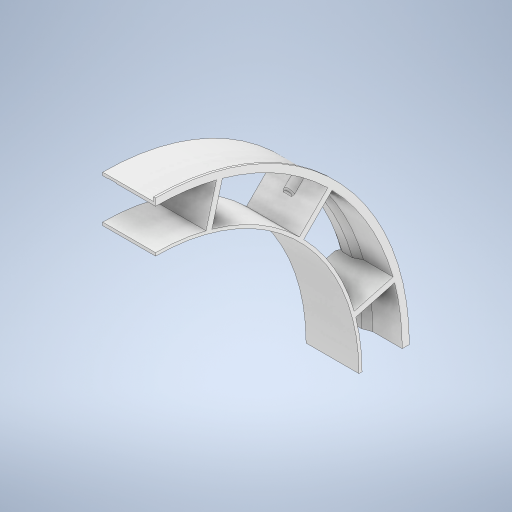
# Autodesk Inventor part: Abstandshalter_Röhre_Neu
Saved by Autodesk Inventor 2023 (Build 270158000, 158)
## iProperties
Created: 2023-03-14
Part Number: Abstandshalter_Röhre_Neu
Material: Generisch
Document SubType Name: Modeling
Designer: prigge
Density: 1 g/cm^3
Appearance: Glatt - Weiß
Author: prigge
Autodesk Inventor part; units mm, degrees
ref_plane "YZ Plane" through (0, 0, 0) normal (1, 0, 0) x (0, 1, 0)
sketch "Skizze1" plane through (0, 0, 0) normal (1, 0, 0) x (0, 1, 0)
  arc A0 (0, -200) -> (200, 0) centre (0, 0) ccw
  arc A1 (0, -203) -> (203, 0) centre (0, 0) ccw
  line L0 (203, 0) -> (200, 0)
  line L1 (0, -200) -> (0, -203)
  line L2 (0, -294.0512) -> (0, 49.0085) projected
  line L3 (-49.0085, 0) -> (294.0512, 0) projected
  dimension "d0" = 200
  dimension "d1" = 3
  constraints: 4 end point, 4 point on circle, 2 centre point, 2 coincident, 2 point on line, 1 horizontal, 1 perpendicular
  measures "d0" radius of A0
  measures "d1" distance of L1.start L1.end
extrude "Extrusion1" add sketch "Skizze1" against normal blind 52 contours A0 L0 A1 L1
sketch "Skizze2" plane through (0, 0, 0) normal (1, 0, 0) x (0, 1, 0)
  arc A0 (0, -242.5) -> (242.5, 0) centre (0, 0) ccw
  arc A1 (0, -245.5) -> (245.5, 0) centre (0, 0) ccw
  line L0 (245.5, 0) -> (242.5, 0)
  line L1 (0, -242.5) -> (0, -245.5)
  line L2 (0, -354.8894) -> (0, 59.1482) projected
  line L3 (-59.1482, 0) -> (354.8894, 0) projected
  dimension "d4" = 3
  dimension "d5" = 245.5
  constraints: 4 end point, 4 point on circle, 2 centre point, 2 coincident, 2 point on line, 1 horizontal, 1 perpendicular
  measures "d4" distance of L1.start L1.end
  measures "d5" radius of A1
extrude "Extrusion2" add sketch "Skizze2" against normal blind 52 contours A0 L0 A1 L1
sketch "Skizze3" plane through (0, 0, 0) normal (1, 0, 0) x (0, 1, 0)
  arc A0 (0, -249.5) -> (249.5, 0) centre (0, 0) ccw
  arc A1 (0, -245.5) -> (245.5, 0) centre (0, 0) ccw projected
  line L0 (242.5, 0) -> (245.5, 0) projected
  arc A2 (0, -245.5) -> (245.5, 0) centre (0, 0) ccw
  line L1 (0, -245.5) -> (0, -249.5)
  line L2 (245.5, 0) -> (249.5, 0)
  dimension "d29" = 4
  constraints: 4 end point, 4 point on circle, 2 centre point, 2 coincident, 1 perpendicular, 1 vertical
  measures "d29" distance of L1.start L1.end
extrude "Extrusion3" add sketch "Skizze3" against normal blind 2
sketch "Skizze4" plane through (0, 0, 0) normal (1, 0, 0) x (0, 1, 0)
  line L0 (0, 0) -> (176.4231, -176.4231) construction
  arc A0 (0, -249.5) -> (249.5, 0) centre (0, 0) ccw projected
  line L1 (0, -362.132) -> (0, 60.3553) projected
  arc A1 (0, -203) -> (203, 0) centre (0, 0) ccw projected
  arc A2 (0, -242.5) -> (242.5, 0) centre (0, 0) ccw projected
  arc A3 (0, -203) -> (203, 0) centre (0, 0) ccw projected
  line L2 (145.6483, -141.4057) -> (173.5816, -169.339)
  arc A4 (0, -242.5) -> (242.5, 0) centre (0, 0) ccw projected
  line L3 (141.4057, -145.6483) -> (169.339, -173.5816)
  point P0 (169.339, -173.5816)
  point P1 (173.5816, -169.339)
  dimension "d11" = 45
  dimension "d12" = 3
  dimension "d13" = 3
  constraints: 6 end point, 5 point on circle
  measures "d11" angle of L1 L0
  measures "d12" distance between parallel lines of L0 L2
  measures "d13" distance between parallel lines of L0 L3
extrude "Extrusion4" add sketch "Skizze4" against normal up to surface (52 mm away) contours L3 A1 L2 A2
pattern_circular "Runde Anordnung1" count 2 over 30 about axis through (-10, 0, 0) along (1, 0, 0) of "Extrusion4"
ref_plane "Arbeitsebene1" through (0, 0, 0) normal (0, 0.7071068, 0.7071068) x (1, 0, 0)
mirror "Spiegeln1" about plane through (0, 0, 0) normal (0, 0.7071068, 0.7071068) of "Extrusion4", "Runde Anordnung1"
ref_plane "Arbeitsebene3" through (0, 171.4734, -171.4734) normal (0, 0.7071068, -0.7071068) x (1, 0, 0)
ref_plane "Arbeitsebene2" through (0, 0, 0) normal (0, 0.7071068, -0.7071068) x (1, 0, 0)
sketch "Skizze5" plane through (0, 171.4734, -171.4734) normal (0, 0.7071068, -0.7071068) x (1, 0, 0)
  circle A0 centre (-27, 0) radius 6
  line L0 (0, 246.9924) -> (0, -246.9924) projected
  circle A1 centre (-27, 0) radius 4
  line L1 (-62.4, 0) -> (10.4, 0) projected
  point P0 (0, 0)
  dimension "d21" = 27
  dimension "d22" = 8
  dimension "d23" = 12
  constraints: 2 centre point, 1 coincident, 1 point on line
  measures "d21" distance from line of L0 A0.centre
  measures "d22" diameter of A1
  measures "d23" diameter of A0
extrude "Extrusion5" add sketch "Skizze5" against normal blind 16
fillet "Rundung2" radius 2 4 edges at (-27, 155.917, -164.4023) (-27, 164.4023, -155.917) (-27, 162.281, -158.0384) (-27, 158.0384, -162.281)
sketch "Skizze9" plane through (0, 0, 0) normal (0, 1, 0) x (-1, 0, 0)
  line L0 (0, -242.5) -> (52, -242.5) projected
  line L1 (52, -245.5) -> (52, -242.5) projected
  line L2 (29, -242.5) -> (37, -239.5)
  line L3 (37, -239.5) -> (47, -239.5)
  line L4 (52, -245.5) -> (52, 0) projected
  line L5 (47, -239.5) -> (47, -242.5)
  line L6 (62.4, 0) -> (-10.4, 0) projected
  point P0 (0, 0)
  dimension "d38" = 3
  dimension "d39" = 5
  dimension "d40" = 18
  dimension "d41" = 10
  constraints: 6 end point, 2 perpendicular, 2 point on line
  measures "d38" distance of L3.end L5.end
  measures "d39" distance between parallel lines of L4 L5
  measures "d40" distance from line of L5 L2.start
  measures "d41" distance of L2.end L3.end
revolve "Umdrehung2" add sketch "Skizze9" angle 87 about axis through (-10, 0, 0) along (1, 0, 0)
sketch "Skizze10" plane through (0, 0, 0) normal (0, 1, 0) x (-1, 0, 0)
  line L0 (47, -242.5) -> (47, -239.5) projected
  line L1 (47, -239.5) -> (37, -239.5) projected
  line L2 (52, -245.5) -> (52, -242.5) projected
  line L3 (47, -240.8) -> (38.5, -240.8)
  line L4 (38.5, -240.8) -> (38.5, -243)
  line L5 (38.5, -243) -> (47, -243)
  line L6 (47, -243) -> (47, -240.8)
  line L7 (47, -242.5) -> (52, -242.5) projected
  line L8 (52, -245.5) -> (52, 0) projected
  arc A0 (47, -240.8) -> (52, -237.0283) centre (47, -235.6) ccw
  line L9 (52, -242.5) -> (52, -237.0283)
  line L10 (63.1578, 0) -> (-10.5263, 0) projected
  line L11 (47, -232.0975) -> (47, -239.5) projected
  point P0 (0, 0)
  dimension "d44" = 2.2
  dimension "d45" = 8.5
  dimension "d46" = 5.2
  dimension "d48" = 0.5
  constraints: 10 end point, 3 point on line, 2 parallel, 2 point on circle, 1 centre point, 1 collinear, 1 horizontal, 1 perpendicular
  measures "d44" distance of L3.end L4.end
  measures "d45" distance of L4.end L5.end
  measures "d46" radius of A0
  measures "d48" distance between parallel lines of L7 L5
revolve "Umdrehung3" cut sketch "Skizze10" angle 90 about axis through (-10, 0, 0) along (1, 0, 0)
fillet "Rundung3" radius 2 1 edges at (-47, 171.8269, -171.8269)
extrude "Extrusion6" cut sketch "Skizze5" along normal mid plane 26 contours L1 A1 | A1 L1
sketch "Skizze7" plane through (0, 0, 0) normal (1, 0, 0) x (0, 1, 0)
  line L0 (0, -242.5) -> (0, -249.5) projected
  circle A0 centre (0, -249.5) radius 2.5
  circle A1 centre (0, -242.5) radius 2.5
  line L1 (0, -203) -> (0, -200) projected
  circle A2 centre (0, -203) radius 2.5
  circle A3 centre (0, -200) radius 2.5
  line L2 (249.5, 0) -> (242.5, 0) projected
  circle A4 centre (249.5, 0) radius 2.5
  circle A5 centre (242.5, 0) radius 2.5
  arc A6 (196.838, -49.6368) -> (203, 0) centre (0, 0) ccw projected
  circle A7 centre (203, 0) radius 2.5
  arc A8 (0, -200) -> (200, 0) centre (0, 0) ccw projected
  circle A9 centre (200, 0) radius 2.5
  point P0 (201.5, -2)
  point P1 (201.5, 2)
  point P2 (2, -201.5)
  point P3 (0, -202.5)
  point P4 (2.5, -199.9844)
  point P5 (-2, -201.5)
  dimension "d35" = 5
  constraints: 8 centre point, 7 equal radius, 3 coincident
  measures "d35" diameter of A1
